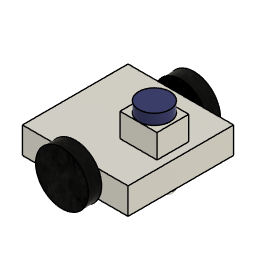
ros2bot (Autodesk Fusion 360 design; units mm, degrees)
Autodesk Fusion 360 part; units mm, degrees
sketch "Sketch1" plane through (0, 0, 0) normal (0, 0, 1) x (1, 0, 0)
sketch "Sketch2" plane through (0, 0, 0) normal (0, 0, 1) x (1, 0, 0)
sketch "Sketch3" plane through (0, 0, 0) normal (0, 0, 1) x (1, 0, 0)
  line L0 (-100, -100) -> (100, -100)
  line L1 (100, -100) -> (100, 100)
  line L2 (100, 100) -> (-100, 100)
  line L3 (-100, 100) -> (-100, -100)
  line L4 (-100, -100) -> (100, 100) construction
  line L5 (100, -100) -> (-100, 100) construction
  dimension "d1" = 200
  dimension "d2" = 200
  constraint horizontal L0
  constraint perpendicular L0 L1
  constraint parallel L0 L2
  constraint parallel L1 L3
  constraint coincident L4 origin
  constraint coincident L5 origin
  measures "d1" distance of L1.end L2.end
  measures "d2" distance of L0.end L1.end
extrude "Extrude1" add sketch "Sketch3" along normal blind 50 makes body 1
sketch "Sketch4" plane through (0, -100, 0) normal (0, -1, 0) x (1, 0, 0)
  line L0 (-100, 0) -> (100, 0)
  line L1 (100, 0) -> (100, 50)
  line L2 (100, 50) -> (-100, 50)
  line L3 (-100, 50) -> (-100, 0)
  circle A0 centre (0, 25) radius 50
  dimension "d5" = 100
  measures "d5" diameter of A0
sketch "Sketch5" plane through (0, 100, 0) normal (0, 1, 0) x (-1, 0, 0)
  line L0 (-100, 0) -> (100, 0)
  line L1 (100, 0) -> (100, 50)
  line L2 (100, 50) -> (-100, 50)
  line L3 (-100, 50) -> (-100, 0)
  circle A0 centre (0, 25) radius 50
  dimension "d6" = 100
  measures "d6" diameter of A0
extrude "Extrude2" add sketch "Sketch4" along normal blind 25 separate body contours L0 L2 A0 | L0 A0 | L2 A0 makes body 2
extrude "Extrude3" add sketch "Sketch5" along normal blind 25 separate body contours L0 L2 A0 | L0 A0 | L2 A0 makes body 3
move_body "Move1" bodies 1 2 3 to x (1, 0, 0) y (0, 1, 0) z (0, 0, 1) at (0, 0, 25)
sketch "Sketch7" plane through (0, 0, 25) normal (0, 0, -1) x (1, 0, 0)
  line L0 (-100, 100) -> (-100, -100)
  line L1 (-100, -100) -> (100, -100)
  line L2 (100, -100) -> (100, 100)
  line L3 (100, 100) -> (-100, 100)
  circle A0 centre (75, 0) radius 12
  dimension "d12" = 24
  measures "d12" diameter of A0
extrude "Extrude4" add sketch "Sketch7" along normal blind 24 contours A0 bodies 1
sketch "Sketch8" plane through (0, 0, 25) normal (0, 0, -1) x (1, 0, 0)
  circle A0 centre (75, 0) radius 12
  line L0 (-100, 100) -> (-100, -100)
  line L1 (-100, -100) -> (100, -100)
  line L2 (100, -100) -> (100, 100)
  line L3 (100, 100) -> (-100, 100)
  circle A1 centre (-75, 0) radius 12
  dimension "d15" = 24
  measures "d15" diameter of A1
extrude "Extrude5" add sketch "Sketch8" along normal blind 24 contours A1 bodies 1
fillet "Fillet1" radius 10 1 faces at (78.1624, 3.7294, 1) on bodies 1
fillet "Fillet2" radius 10 1 faces at (-82.4167, -0.8556, 1) on bodies 1
sketch "Sketch9" plane through (0, 0, 75) normal (0, 0, 1) x (-1, 0, 0)
  line L0 (100, -100) -> (100, 100)
  line L1 (100, 100) -> (-100, 100)
  line L2 (-100, 100) -> (-100, -100)
  line L3 (-100, -100) -> (100, -100)
  line L4 (-15, -30) -> (-85, -30)
  line L5 (-85, -30) -> (-85, 30)
  line L6 (-85, 30) -> (-15, 30)
  line L7 (-15, 30) -> (-15, -30)
  line L8 (-15, -30) -> (-85, 30) construction
  line L9 (-85, -30) -> (-15, 30) construction
  point P0 (-50, 0)
  dimension "d22" = 70
  dimension "d23" = 60
  constraint horizontal L4
  constraint perpendicular L4 L5
  constraint parallel L4 L6
  constraint parallel L5 L7
  constraint coincident L8 P0
  constraint coincident L9 P0
  measures "d22" distance of L5.end L6.end
  measures "d23" distance of L4.end L5.end
extrude "Extrude6" add sketch "Sketch9" along normal blind 45 contours L4 L5 L6 L7 bodies 1
sketch "Sketch10" plane through (0, 0, 120) normal (0, 0, 1) x (-1, 0, 0)
  line L0 (-15, 30) -> (-85, 30)
  line L1 (-85, 30) -> (-85, -30)
  line L2 (-85, -30) -> (-15, -30)
  line L3 (-15, -30) -> (-15, 30)
  circle A0 centre (-50, 0) radius 29.5
  dimension "d26" = 59
  measures "d26" diameter of A0
extrude "Extrude7" add sketch "Sketch10" along normal blind 20 separate body contours A0 makes body 4
copy_body "Body->Comp1" bodies 1 removing the originals makes body 5 in component "base_link"
copy_body "Body->Comp2" bodies 2 removing the originals makes body 6 in component "right_wheel"
copy_body "Body->Comp3" bodies 3 removing the originals makes body 7 in component "left_wheel"
copy_body "Body->Comp4" bodies 4 removing the originals makes body 8 in component "lidar"
component "base_link" placed x (1, 0, 0) y (0, 1, 0) z (0, 0, 1) at (0, 0, 0)
component "right_wheel" placed x (1, 0, 0) y (0, 1, 0) z (0, 0, 1) at (0, 0, 0)
component "left_wheel" placed x (1, 0, 0) y (0, 1, 0) z (0, 0, 1) at (0, 0, 0)
component "lidar" placed x (1, 0, 0) y (0, 1, 0) z (0, 0, 1) at (0, 0, 0)
named bodies: "base_link", "right_wheel", "left_wheel", "lidar"
